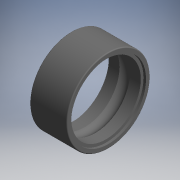
# Autodesk Inventor part: 684AZZ Outer Ring
Saved by Autodesk Inventor 2017.3 (Build 213256000, 256)
## iProperties
Part Number: 684AZZ Outer Ring
Material: Generic
Catalog Web Link: www.cadenas.de
Description: shielde_type_zz_zzs_OR-
Vendor: NSK_RB
Document SubType Name: Modeling
Designer: partserver
Manufacturer: NSK_RB
Mass: 0.0690437 g
Surface Area: 2.49476 cm^2
Volume: 0.0690437 cm^3
Density: 1 g/cm^3
Appearance: PSOLRGB-128-128-128
Category: PARTsolutions
Company: NSK_RB
Title: 684AZZ Outer Ring
Author: Cadenas PARTsolutions
PSOL_IDENT_0: {$CADENAS_DATA\23d-libs\nsk_rb\roller_bearings\deep_groove_bb\exstra_small_miniatur_bb\metric_design
PSOL_IDENT_1: \shielded_type_zz_zzs_or.prj},191 {VTYP=3D},{NB=684AZZ Outer Ring},{LINA=684AZZ Outer Ring},{NN=shie
PSOL_IDENT_2: lde_type_zz_zzs_OR},{DATE=30.03.2022 01:55:07},{GEOMDATE=04.01.2008 00:00:00},{VERSION=},{LINEID=220
PSOL_IDENT_3: },{WBVAR=},{WBNUMERIC=}  {NB=684AZZ Outer Ring},{LINA=684AZZ Outer Ring},{KT=DUMMY},{IDNR=},{STAN=St
PSOL_IDENT_4: andard},{ORDER=684AZZ},{SD=4.0},{X=4.0},{DI1=5.20},{DI2=5.20},{SDE1=7.50},{SDE2=8.10},{D=9},{DD=9},{
PSOL_IDENT_5: B=2.5},{B1=4.0},{R=0.10},{R1=0.10},{CR1=640},{COR1=225},{CR2=65},{COR2=23.0},{LG=53000},{LO=63000},{
PSOL_IDENT_6: DA=0.0},{DB=5.2},{DA1=0.0},{DB1=8.1},{RA=0.00},{RB=0.10},{MASS=1.01},{SC=1}
NB: 684AZZ Outer Ring
NN: shielde_type_zz_zzs_OR
NBSYN: $ORDER. Outer Ring
LINA: 684AZZ Outer Ring
CATALOG: NSK Rolling Bearing
STAN: Standard
ORDER: 684AZZ
SD: 4
X: 4
DI1: 5.2
DI2: 5.2
SDE1: 7.5
SDE2: 8.1
D: 9
DD: 9
B: 2.5
B1: 4
R: 0.1
R1: 0.1
CR1: 640
COR1: 225
CR2: 65
COR2: 23
LG: 53000
LO: 63000
DA: 0
DB: 5.2
DA1: 0
DB1: 8.1
RA: 0
RB: 0.1
MASS: 1.01
SC: 1
SUPPLIER: NSK_RB
ARTICLENO: 684AZZ Outer Ring
BOMINFO: 684AZZ Outer Ring
CREATOR: CADENAS GmbH
Autodesk Inventor part; units mm, degrees
sketch "Sketch_1" plane through (0, 0, 0) normal (0, 0, 1) x (1, 0, 0)
  line L0 (4, 0) -> (0, 0)
  line L1 (0, 4.05) -> (0.2656, 4.05)
  line L2 (0.2656, 4.05) -> (0.2656, 3.75)
  line L3 (0.2656, 3.75) -> (1.441, 3.75)
  arc A0 (2.559, 3.75) -> (1.441, 3.75) centre (2, 3.25) ccw
  line L4 (2.559, 3.75) -> (3.7344, 3.75)
  line L5 (3.7344, 3.75) -> (3.7344, 4.05)
  line L6 (3.7344, 4.05) -> (4, 4.05)
  line L7 (4, 4.05) -> (4, 4.4)
  arc A1 (4, 4.4) -> (3.9, 4.5) centre (3.9, 4.4) ccw
  line L8 (3.9, 4.5) -> (0.1, 4.5)
  arc A2 (0.1, 4.5) -> (0, 4.4) centre (0.1, 4.4) ccw
  line L9 (0, 4.4) -> (0, 4.05)
  constraints: 20 end point, 6 point on circle, 3 centre point
revolve "Revolution1" add sketch "Sketch_1" angle 360 about axis through (4, 0, 0) along (1, 0, 0)
ref_plane "ip_st_or_1_XY" through (0, 0, 0) normal (1, 0, 0) x (0, 0, -1)
ref_plane "ip_st_or_1_YZ" through (0, 0, 0) normal (0, 0, -1) x (0, 1, 0)
ref_plane "ip_st_or_1_ZX" through (0, 0, 0) normal (0, 1, 0) x (1, 0, 0)
ref_plane "ip_st_or_2_XY" through (3.7344, 0, 0) normal (-1, 0, 0) x (0, 0, -1)
ref_plane "ip_st_or_2_YZ" through (3.7344, 0, 0) normal (0, 0, -1) x (0, -1, 0)
ref_plane "ip_st_or_2_ZX" through (3.7344, 0, 0) normal (0, -1, 0) x (-1, 0, 0)
body "Solid1"
